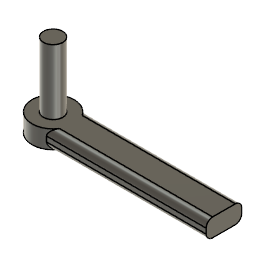
Ball launcher (Autodesk Fusion 360 archive; units mm, degrees)
design "Slider & Revolute joint"
Autodesk Fusion 360 part; units mm, degrees
sketch "Sketch1" plane through (0, 0, 0) normal (0, 0, 1) x (1, 0, 0)
  line L0 (1.7321, 2.75) -> (26.3431, 2.75)
  line L1 (26.3431, 2.75) -> (26.3431, -2.75)
  line L2 (26.3431, -2.75) -> (1.7321, -2.75)
  arc A0 (1.7321, 2.75) -> (1.7321, -2.75) centre (0, 0) ccw
  dimension "d1" = 6.5
  dimension "d2" = 5.5
  dimension "d3" = 24.611
  dimension "d4" = 5.5
  constraint coincident A0.centre origin
  constraint perpendicular L0 L1
  measures "d1" diameter of A0
  measures "d2" distance of L0.start L2.end
  measures "d3" distance of L0.start L0.end
  measures "d4" distance of L0.end L1.end
sketch "Sketch2" plane through (0, 0, 0) normal (0, 0, 1) x (1, 0, 0)
sketch "Sketch3" plane through (0, 0, 0) normal (0, 0, 1) x (1, 0, 0)
extrude "Extrude1" add sketch "Sketch1" along normal blind 2.8
sketch "Sketch4" plane through (0, 0, 2.8) normal (0, 0, 1) x (-1, 0, 0)
  line L0 (-26.3431, -2.75) -> (-1.7321, -2.75)
  arc A0 (-1.7321, -2.75) -> (-1.7321, 2.75) centre (0, 0) ccw
  line L1 (-1.7321, 2.75) -> (-26.3431, 2.75)
  line L2 (-26.3431, 2.75) -> (-26.3431, -2.75)
  circle A1 centre (0, 0) radius 1.5
  dimension "d7" = 3
  constraint concentric A0 A1
  measures "d7" diameter of A1
extrude "Extrude2" add sketch "Sketch4" along normal blind 10 contours A1
fillet "Fillet1" radius 1 4 edges at (14.0376, -2.75, 2.8) (14.0376, 2.75, 2.8) (14.0376, 2.75, 0) (14.0376, -2.75, 0)

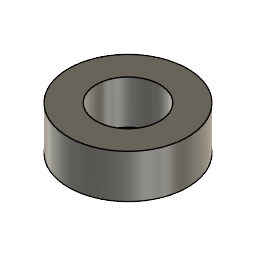
design "Washer"
Autodesk Fusion 360 part; units mm, degrees
sketch "Sketch1" plane through (0, 0, 0) normal (0, 0, 1) x (1, 0, 0)
  circle A0 centre (0, 0) radius 3
  dimension "d1" = 6
  constraint coincident A0.centre origin
  measures "d1" diameter of A0
extrude "Extrude1" add sketch "Sketch1" along normal blind 2.2
hole "Hole1" at (0, 0, 2.2) direction (0, 0, -1) diameter 3.2 depth 101.732 tip angle 118

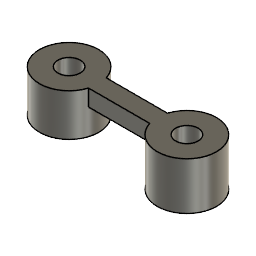
design "Linkers"
Autodesk Fusion 360 part; units mm, degrees
sketch "Sketch1" plane through (0, 0, 0) normal (0, 0, 1) x (1, 0, 0)
  circle A0 centre (0, 0) radius 4.5
  line L0 (0, 0) -> (17.87, 0) construction
  circle A1 centre (17.87, 0) radius 4.5
  line L1 (13.5773, 1.35) -> (4.2927, 1.35)
  line L2 (13.5773, -1.35) -> (4.2927, -1.35)
  dimension "d1" = 9
  dimension "d2" = 17.87
  dimension "d3" = 9
  dimension "d4" = 2.7
  dimension "d5" = 1.35
  constraint coincident A0.centre L0.start
  constraint horizontal L0
  constraint coincident L0.end A1.centre
  constraint coincident A1 L1.start
  constraint coincident A0 L1.end
  constraint horizontal L1
  constraint coincident A1 L2.start
  constraint coincident A0 L2.end
  constraint parallel L0 L2
  measures "d1" diameter of A0
  measures "d2" distance of A0.centre L0.end
  measures "d3" diameter of A1
  measures "d4" distance of L1 L2
  measures "d5" distance of L0 L1
extrude "Extrude1" add sketch "Sketch1" along normal blind 6.4 contours A0 makes body 1
sketch "Sketch2" plane through (0, 0, 6.4) normal (0, 0, 1) x (-1, 0, 0)
  circle A0 centre (0, 0) radius 4.5
  line L0 (0, 0) -> (-17.87, 0) construction
  circle A1 centre (-17.87, 0) radius 4.5
  dimension "d8" = 17.87
  dimension "d9" = 9
  constraint coincident A0.centre L0.start
  constraint horizontal L0
  constraint coincident L0.end A1.centre
  measures "d8" distance of A0.centre L0.end
  measures "d9" diameter of A1
extrude "Extrude2" add sketch "Sketch2" against normal blind 7.2 separate body contours A1 makes body 2
sketch "Sketch3" plane through (0, 0, 6.4) normal (0, 0, 1) x (-1, 0, 0)
  circle A0 centre (0, 0) radius 4.5
  circle A1 centre (0, 0) radius 4.5
  line L0 (0, 0) -> (-17.87, 0) construction
  circle A2 centre (-17.87, 0) radius 4.5
  line L1 (-4.2925, -1.3507) -> (-13.5775, -1.3507)
  line L2 (-13.5775, 1.3507) -> (-4.2925, 1.3507)
  dimension "d12" = 17.87
  dimension "d13" = 9
  dimension "d14" = 9.285
  dimension "d15" = 9.285
  constraint coincident A0.centre A1.centre
  constraint horizontal L0
  constraint coincident L0.end A2.centre
  constraint coincident A1 L1.start
  constraint coincident A2 L1.end
  constraint parallel L0 L1
  constraint coincident A2 L2.start
  constraint coincident A1 L2.end
  constraint horizontal L2
  measures "d12" distance of A0.centre L0.end
  measures "d13" diameter of A2
  measures "d14" distance of L1.start L1.end
  measures "d15" distance of L2.start L2.end
extrude "Extrude3" add sketch "Sketch3" against normal blind 2.49 contours A0 A1 A2 L1 L2 bodies 1 2
sketch "Sketch4" plane through (0, 0, 0) normal (0, 1, 0) x (1, 0, 0)
hole "Hole1" at (0, 0, 6.4) direction (0, 0, -1) diameter 3.4 depth 7 tip angle 118 bodies 1
hole "Hole2" at (17.87, 0, 6.4) direction (0, 0, -1) diameter 3.4 depth 7 tip angle 118 bodies 1

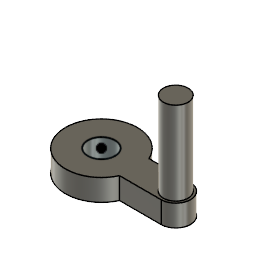
design "Grank"
Autodesk Fusion 360 part; units mm, degrees
sketch "Sketch5" plane through (0, 0, 0) normal (0, 0, 1) x (1, 0, 0)
  line L0 (9.3481, 1.8494) -> (4.1024, 1.8494)
  line L1 (9.3481, -1.8494) -> (4.1024, -1.8494)
  arc A0 (9.2519, -1.8494) -> (9.2519, 1.8494) centre (9.3, 0) ccw
  arc A1 (4.1024, 1.8494) -> (4.1024, -1.8494) centre (0, 0) ccw
  dimension "d23" = 9
  dimension "d24" = 3.7
  dimension "d25" = 9.3
  constraint coincident A1.centre origin
  constraint coincident L0.start A0
  constraint horizontal L0
  constraint coincident L1.start A0
  constraint parallel L0 L1
  constraint coincident L0 A0.end
  constraint coincident L1 A0.start
  measures "d23" diameter of A1
  measures "d24" diameter of A0
  measures "d25" distance of A1.centre A0.centre
sketch "Sketch6" plane through (0, 0, 0) normal (0, 0, 1) x (1, 0, 0)
  circle A0 centre (0, 0) radius 1.7
  dimension "d26" = 3.4
  constraint coincident A0.centre origin
  measures "d26" diameter of A0
extrude "Extrude6" add sketch "Sketch5" against normal blind 2.7
hole "Hole2" at (0, 0, 0) direction (0, 0, -1) diameter 3.4 depth 2.7 tip angle 118
sketch "Sketch7" plane through (0, 0, 0) normal (0, 0, 1) x (1, 0, 0)
  circle A0 centre (9.3, 0) radius 1.55
  dimension "d32" = 3.1
  dimension "d33" = 9.3
  measures "d32" diameter of A0
  measures "d33" distance of A0.centre origin
extrude "Extrude7" add sketch "Sketch7" along normal blind 10.4
sketch "Sketch1" plane through (0, 0, 0) normal (0, 0, 1) x (1, 0, 0)
  circle A0 centre (0, 0) radius 10.7065
  dimension "d1" = 21.413
  constraint coincident A0.centre origin
  measures "d1" diameter of A0
extrude "Extrude1" [rolled back] along distance -1.943 taper angle 0
sketch "Sketch2" plane through (0, 0, 0) normal (0, 0, 1) x (1, 0, 0)
  circle A0 centre (0, 0) radius 1.5
  dimension "d4" = 3
  constraint coincident A0.centre origin
  measures "d4" diameter of A0
sketch "Sketch3" plane through (0, 0, 0) normal (0, 0, 1) x (1, 0, 0)
  circle A0 centre (0, 0) radius 1.5
  circle A1 centre (7.5, 0) radius 1.5
  dimension "d7" = 3
  dimension "d9" = 3
  dimension "d10" = 7.5
  constraint coincident A0.centre origin
  measures "d7" diameter of A0
  measures "d9" diameter of A1
  measures "d10" distance of A0.centre A1.centre
sketch "Sketch4" plane through (0, 0, 0) normal (0, 0, 1) x (1, 0, 0)
  circle A0 centre (0, 0) radius 1.5
  dimension "d8" = 3
  constraint coincident A0.centre origin
  measures "d8" diameter of A0
extrude "Extrude3" [rolled back] side1wall thickness 0.1 along distance 2.8 taper angle 0
hole "Hole1" [rolled back] hole depth 2.5 hole diameter 2.305 tip angle 118
extrude "Extrude4" [rolled back] side1wall thickness 0.348 along distance 7 taper angle 0
extrude "Extrude5" [rolled back] side1wall thickness 0.348 along distance 2.8 taper angle 0
split "Split1" [rolled back]

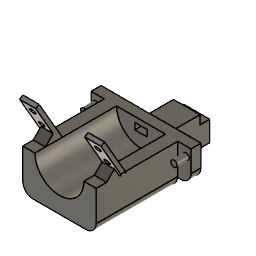
design "Mount for ball feeder"
Autodesk Fusion 360 part; units mm, degrees
sketch "Sketch1" plane through (0, 0, 0) normal (0, 0, 1) x (1, 0, 0)
sketch "Sketch2" plane through (0, 0, 0) normal (0, 0, 1) x (1, 0, 0)
  line L0 (0, 0) -> (13, 0)
  line L1 (13, 0) -> (13, 14.337)
  line L2 (13, 14.337) -> (0, 14.337)
  line L3 (0, 14.337) -> (0, 0)
  dimension "d1" = 13
  dimension "d2" = 14.337
  constraint horizontal L0
  constraint vertical L1
  constraint horizontal L2
  constraint vertical L3
  constraint coincident L0.start L3.end
  measures "d1" distance of L0.start L0.end
  measures "d2" distance of L0.start L2.end
extrude "Extrude1" add sketch "Sketch2" along normal blind 27.237
sketch "Sketch3" plane through (13, 0, 0) normal (1, 0, 0) x (0, 1, 0)
  line L0 (0, 0) -> (14.337, 0)
  line L1 (14.337, 0) -> (14.337, 27.237)
  line L2 (14.337, 27.237) -> (0, 27.237)
  line L3 (0, 27.237) -> (0, 0)
  line L4 (0, 27.237) -> (4.337, 27.237)
  line L5 (4.337, 27.237) -> (4.337, 22.419)
  line L6 (4.337, 22.419) -> (0, 22.419)
  line L7 (0, 22.419) -> (0, 27.237)
  dimension "d5" = 4.818
  dimension "d6" = 4.337
  constraint horizontal L4
  constraint vertical L5
  constraint horizontal L6
  constraint vertical L7
  constraint coincident L2.end L3.start
  measures "d5" distance of L2.end L6.end
  measures "d6" distance of L2.end L4.end
extrude "Extrude2" cut sketch "Sketch3" against normal blind 100 contours L2 L3 L4 L5 L6 L7
sketch "Sketch4" plane through (0, 0, 22.419) normal (0, 0, 1) x (-1, 0, 0)
  line L0 (0, -4.337) -> (0, 0)
  line L1 (0, 0) -> (-13, 0)
  line L2 (-13, 0) -> (-13, -4.337)
  line L3 (-13, -4.337) -> (0, -4.337)
sketch "Sketch5" plane through (0, 0, 0) normal (0, 0, 1) x (1, 0, 0)
  line L0 (0, 0) -> (13, 0)
  line L1 (13, 0) -> (13, -5.663)
  line L2 (13, -5.663) -> (0, -5.663)
  line L3 (0, -5.663) -> (0, 0)
  dimension "d9" = 5.663
  constraint horizontal L0
  constraint vertical L1
  constraint horizontal L2
  constraint vertical L3
  constraint coincident L0.start L3.end
  measures "d9" distance of L0.start L2.end
extrude "Extrude3" add sketch "Sketch5" along normal blind 4.919
sketch "Sketch6" plane through (0, 0, 4.919) normal (0, 0, 1) x (-1, 0, 0)
  line L0 (0, 5.663) -> (-13, 5.663)
  line L1 (-13, 5.663) -> (-13, 0)
  line L2 (-13, 0) -> (0, 0)
  line L3 (0, 0) -> (0, 5.663)
  line L4 (-3.5, 0) -> (-9.5, 0)
  line L5 (-9.5, 0) -> (-9.5, 3.168)
  line L6 (-9.5, 3.168) -> (-3.5, 3.168)
  line L7 (-3.5, 3.168) -> (-3.5, 0)
  dimension "d12" = 6
  dimension "d13" = 3.168
  dimension "d14" = 3.5
  constraint horizontal L4
  constraint vertical L5
  constraint horizontal L6
  constraint vertical L7
  constraint coincident L2 L4.start
  measures "d12" distance of L4.start L4.end
  measures "d13" distance of L4.start L6.end
  measures "d14" distance of L3 L7
extrude "Extrude4" cut sketch "Sketch6" against normal blind 10 contours L2 L4 L5 L6 L7
sketch "Sketch7" plane through (13, 0, 0) normal (1, 0, 0) x (0, 1, 0)
  line L0 (4.337, 22.419) -> (0, 22.419)
  line L1 (0, 22.419) -> (0, 4.919)
  line L2 (0, 4.919) -> (-5.663, 4.919)
  line L3 (-5.663, 4.919) -> (-5.663, 0)
  line L4 (-5.663, 0) -> (14.337, 0)
  line L5 (14.337, 0) -> (14.337, 27.237)
  line L6 (14.337, 27.237) -> (4.337, 27.237)
  line L7 (4.337, 27.237) -> (4.337, 22.419)
  line L8 (-5.663, 4.919) -> (9.837, 4.919)
  line L9 (9.837, 4.919) -> (9.837, 0)
  line L10 (9.837, 0) -> (-5.663, 0)
  line L11 (-5.663, 0) -> (-5.663, 4.919)
  dimension "d17" = 15.5
  constraint horizontal L8
  constraint vertical L9
  constraint horizontal L10
  constraint vertical L11
  constraint coincident L2.end L3.start
  measures "d17" distance of L2.end L8.end
extrude "Extrude5" add sketch "Sketch7" along normal blind 18 contours L2 L3 L4 L8 L9 L10 L11
sketch "Sketch8" plane through (0, 0, 0) normal (-1, 0, 0) x (0, -1, 0)
  line L0 (0, 22.419) -> (-4.337, 22.419)
  line L1 (-4.337, 22.419) -> (-4.337, 27.237)
  line L2 (-4.337, 27.237) -> (-14.337, 27.237)
  line L3 (-14.337, 27.237) -> (-14.337, 0)
  line L4 (-14.337, 0) -> (5.663, 0)
  line L5 (5.663, 0) -> (5.663, 4.919)
  line L6 (5.663, 4.919) -> (0, 4.919)
  line L7 (0, 4.919) -> (0, 22.419)
  line L8 (5.663, 4.919) -> (-9.837, 4.919)
  line L9 (-9.837, 4.919) -> (-9.837, 0)
  line L10 (-9.837, 0) -> (5.663, 0)
  line L11 (5.663, 0) -> (5.663, 4.919)
  dimension "d20" = 15.5
  constraint horizontal L8
  constraint vertical L9
  constraint horizontal L10
  constraint vertical L11
  constraint coincident L5.end L6.start
  measures "d20" distance of L5.end L8.end
extrude "Extrude6" add sketch "Sketch8" along normal blind 18 contours L4 L5 L6 L8 L9 L10 L11
fillet "Fillet1" radius 5 2 edges at (31, 9.837, 2.4595) (-18, 9.837, 2.4595)
sketch "Sketch9" plane through (0, 0, 0) normal (0, 0, -1) x (1, 0, 0)
  line L0 (9.5, 3.168) -> (9.5, 0)
  line L1 (9.5, 0) -> (3.5, 0)
  line L2 (3.5, 0) -> (3.5, 3.168)
  line L3 (3.5, 3.168) -> (9.5, 3.168)
  arc A0 (-18, -4.837) -> (-13, -9.837) centre (-13, -4.837) ccw
  line L4 (-13, -9.837) -> (0, -9.837)
  line L5 (0, -9.837) -> (0, -14.337)
  line L6 (0, -14.337) -> (13, -14.337)
  line L7 (13, -14.337) -> (13, -9.837)
  line L8 (13, -9.837) -> (26, -9.837)
  arc A1 (26, -9.837) -> (31, -4.837) centre (26, -4.837) ccw
  line L9 (31, -4.837) -> (31, 5.663)
  line L10 (31, 5.663) -> (-18, 5.663)
  line L11 (-18, 5.663) -> (-18, -4.837)
  circle A2 centre (-15.644, 1.274) radius 1.5
  dimension "d25" = 3
  dimension "d26" = 4.389
  dimension "d27" = 2.356
  measures "d25" diameter of A2
  measures "d26" distance of L10 A2.centre
  measures "d27" distance of L11 A2.centre
sketch "Sketch10" plane through (0, 0, 0) normal (0, 0, -1) x (1, 0, 0)
  circle A0 centre (28.644, 1.274) radius 1.5
  line L0 (31, 5.663) -> (-18, 5.663)
  line L1 (31, -4.837) -> (31, 5.663)
  dimension "d28" = 3
  dimension "d29" = 4.389
  dimension "d30" = 2.356
  measures "d28" diameter of A0
  measures "d29" distance of A0.centre L0
  measures "d30" distance of A0.centre L1
extrude "Extrude7" add sketch "Sketch10" sketch "Sketch9" along normal blind 6 of sketch 2 contours A2
sketch "Sketch11" plane through (0, 0, 0) normal (0, 0, -1) x (1, 0, 0)
  circle A0 centre (-15.644, 1.274) radius 1.5
  circle A1 centre (28.644, 1.274) radius 1.5
  line L0 (9.5, 3.168) -> (9.5, 0)
  line L1 (9.5, 0) -> (3.5, 0)
  line L2 (3.5, 0) -> (3.5, 3.168)
  line L3 (3.5, 3.168) -> (9.5, 3.168)
  arc A2 (-18, -4.837) -> (-13, -9.837) centre (-13, -4.837) ccw
  line L4 (-13, -9.837) -> (0, -9.837)
  line L5 (0, -9.837) -> (0, -14.337)
  line L6 (0, -14.337) -> (13, -14.337)
  line L7 (13, -14.337) -> (13, -9.837)
  line L8 (13, -9.837) -> (26, -9.837)
  arc A3 (26, -9.837) -> (31, -4.837) centre (26, -4.837) ccw
  line L9 (31, -4.837) -> (31, 5.663)
  line L10 (31, 5.663) -> (-18, 5.663)
  line L11 (-18, 5.663) -> (-18, -4.837)
  line L12 (-11.5, 5.663) -> (24.5, 5.663)
  line L13 (24.5, 5.663) -> (24.5, -14.337)
  line L14 (24.5, -14.337) -> (-11.5, -14.337)
  line L15 (-11.5, -14.337) -> (-11.5, 5.663)
  dimension "d33" = 36
  dimension "d34" = 20
  dimension "d35" = 6.5
  constraint horizontal L12
  constraint vertical L13
  constraint horizontal L14
  constraint vertical L15
  constraint coincident L10 L12.start
  measures "d33" distance of L12.start L12.end
  measures "d34" distance of L12.start L14.end
  measures "d35" distance of L11 L15
extrude "Extrude8" add sketch "Sketch11" along normal blind 40 contours L0 L1 L2 L3 | L4 L5 L6 L7 L8 L10 L12 L13 L14 L15 | L4 L5 L14 L15 | L7 L8 L13 L14
sketch "Sketch12" plane through (0, 0, -40) normal (0, 0, -1) x (1, 0, 0)
  line L0 (-11.5, -14.337) -> (24.5, -14.337)
  line L1 (24.5, -14.337) -> (24.5, 5.663)
  line L2 (24.5, 5.663) -> (-11.5, 5.663)
  line L3 (-11.5, 5.663) -> (-11.5, -14.337)
  circle A0 centre (6.5, 5.663) radius 12
  dimension "d38" = 24
  constraint midpoint L2 A0.centre
  measures "d38" diameter of A0
extrude "Extrude9" cut sketch "Sketch12" against normal blind 40 contours L2 A0 picked at (8.994, 2.5357)
fillet "Fillet2" radius 5 2 edges at (24.5, 14.337, -20) (-11.5, 14.337, -20)
sketch "Sketch13" plane through (-11.5, 0, 0) normal (-1, 0, 0) x (0, -1, 0)
  line L0 (-9.337, 0) -> (-9.337, -40)
  line L1 (-9.337, -40) -> (5.663, -40)
  line L2 (5.663, -40) -> (5.663, 0)
  line L3 (5.663, 0) -> (-9.337, 0)
  line L4 (5.663, 0) -> (5.663, -26.552)
  line L5 (5.663, -26.552) -> (25.3192, -37.9005)
  line L6 (5.663, -26.552) -> (28.36, -26.552) construction
  line L7 (25.3192, -37.9005) -> (24.3192, -39.6326)
  line L8 (24.3192, -39.6326) -> (5.663, -28.8614)
  line L9 (5.663, -28.8614) -> (5.663, -26.552)
  dimension "d43" = 26.552
  dimension "d44" = 30
  dimension "d45" = 22.697
  dimension "d46" = 2
  constraint coincident L2.end L3.start
  constraint coincident L2 L4.end
  constraint horizontal L6
  constraint perpendicular L5 L7
  constraint coincident L2 L8.end
  constraint perpendicular L7 L8
  measures "d43" distance of L2.end L4.end
  measures "d44" angle of L5 L6
  measures "d45" distance of L4.end L5.end
  measures "d46" distance of L5.end L7.end
extrude "Extrude10" add sketch "Sketch13" against normal blind 6 contours L2 L5 L7 L8 L9
sketch "Sketch14" plane through (-11.5, 0, 0) normal (-1, 0, 0) x (0, -1, 0)
  line L0 (-9.337, 0) -> (-9.337, -40)
  line L1 (-9.337, -40) -> (5.663, -40)
  line L2 (5.663, -40) -> (5.663, -28.8614)
  line L3 (5.663, -28.8614) -> (24.3192, -39.6326)
  line L4 (24.3192, -39.6326) -> (25.3192, -37.9005)
  line L5 (25.3192, -37.9005) -> (5.663, -26.552)
  line L6 (5.663, -26.552) -> (5.663, 0)
  line L7 (5.663, 0) -> (-9.337, 0)
  line L8 (5.663, -26.552) -> (5.663, -28.8614)
  line L9 (5.663, -28.8614) -> (24.3192, -39.6326)
  line L10 (25.3192, -37.9005) -> (5.663, -26.552)
  constraint coincident L5.end L6.start
  constraint coincident L2.end L3.start
  constraint coincident L3.end L4.start
  constraint coincident L4.end L5.start
extrude "Extrude11" add sketch "Sketch14" along normal blind 2 contours L3 L4 L5 L8 L9 L10
fillet "Fillet3" radius 2 1 edges at (-13.5, -5.663, -27.7067)
sketch "Sketch15" plane through (0, 10.0816, -17.4618) normal (0, -0.5, 0.866025) x (1, 0, 0)
  ellipse E0 centre (-11.5, -20.4897) end of major axis (-11.5, -18.1803) minor radius 2 (-11.5, -18.1803) -> (-13.5, -20.4897) ccw
  line L0 (-13.5, -20.4897) -> (-13.5, -40.8773)
  line L1 (-13.5, -40.8773) -> (-5.5, -40.8773)
  line L2 (-5.5, -40.8773) -> (-5.5, -18.1803)
  line L3 (-5.5, -18.1803) -> (-11.5, -18.1803)
  circle A0 centre (-9.5, -35.8803) radius 1.5
  circle A1 centre (-9.5, -26.8803) radius 1.5
  dimension "d53" = 3
  dimension "d54" = 4
  dimension "d55" = 3
  dimension "d56" = 8.7
  dimension "d57" = 4
  dimension "d58" = 9
  measures "d53" diameter of A0
  measures "d54" distance of L2 A0.centre
  measures "d55" diameter of A1
  measures "d56" distance of L3 A1.centre
  measures "d57" distance of L2 A1.centre
  measures "d58" distance of A0.centre A1.centre
extrude "Extrude12" cut sketch "Sketch15" against normal blind 10 contours A0 | A1
sketch "Sketch16" plane through (-11.5, 0, 0) normal (-1, 0, 0) x (0, -1, 0)
  line L0 (5.663, -28.8614) -> (5.663, -26.552)
  line L1 (5.663, -26.552) -> (5.663, 0)
  line L2 (5.663, 0) -> (-9.337, 0)
  line L3 (-9.337, 0) -> (-9.337, -40)
  line L4 (-9.337, -40) -> (5.663, -40)
  line L5 (5.663, -40) -> (5.663, -28.8614)
  line L6 (5.663, -28.8614) -> (5.663, -34.8614)
  line L7 (5.663, -28.8614) -> (20.746, -37.5696) construction
  line L8 (5.663, -28.8614) -> (23.0793, -28.8614) construction
  line L9 (5.663, -34.8614) -> (9.4668, -31.0576)
  line L10 (5.663, -34.8614) -> (11.0425, -34.8614) construction
  line L11 (9.4668, -31.0576) -> (5.663, -28.8614)
  dimension "d61" = 6
  dimension "d62" = 30
  dimension "d63" = 45
  constraint coincident L0.start L5.end
  constraint parallel L5 L6
  constraint horizontal L8
  constraint horizontal L10
  constraint coincident L7 L9.end
  measures "d61" distance of L0.start L6.end
  measures "d62" angle of L7 L8
  measures "d63" angle of L9 L10
extrude "Extrude13" add sketch "Sketch16" against normal blind 6 contours L5 L6 L9 L11
ref_plane "WorkPlane1" through (6.5, 7.1685, 13.6185) normal (-1, 0, 0) x (0, -1, 0)
mirror "Mirror1" about plane through (6.5, 7.1685, 13.6185) normal (-1, 0, 0) of bodies 1 merged
move_body "Move1" bodies 1 to x (1, 0, 0) y (0, 1, 0) z (0, 0, 1) at (-6.5, -14.337, -27.237)
move_body "Move2" bodies 1 to x (1, 0, 0) y (0, 0, -1) z (0, 1, 0) at (0, 0, 0)
